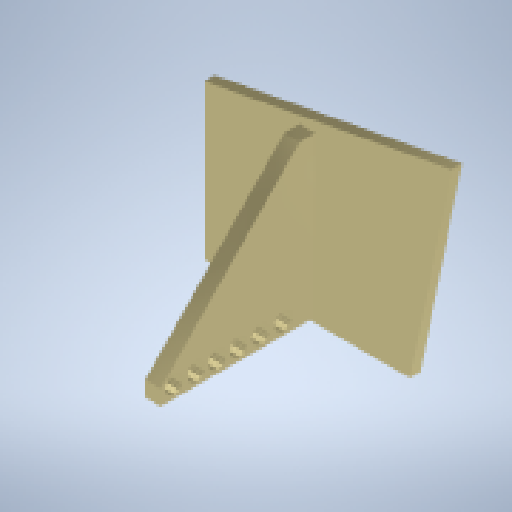
# Autodesk Inventor part: Part5
Saved by Autodesk Inventor 2025.3 (Build 293356000, 356)
## iProperties
Created: 2025-07-14
Part Number: Part5
Material: Generic
Document SubType Name: Modeling
Designer: steve
Density: 1 g/cm^3
Appearance: Default
Author: steve
Autodesk Inventor part; units mm, degrees
ref_plane "YZ Plane" through (0, 0, 0) normal (1, 0, 0) x (0, 1, 0)
ref_plane "XZ Plane" through (0, 0, 0) normal (0, 1, 0) x (-1, 0, 0)
ref_plane "XY Plane" through (0, 0, 0) normal (0, 0, 1) x (1, 0, 0)
sketch "Sketch1" plane through (0, 0, 0) normal (0, 0, 1) x (1, 0, 0)
  line L0 (12.5729, -9.5) -> (10, -7.5)
  line L1 (10, -7.5) -> (-10, -7.5)
  line L2 (-10, -7.5) -> (-10, 7.5)
  line L3 (10, -7.5) -> (14.037, 12.0883)
  line L4 (14.037, 12.0883) -> (-10, 7.5)
  point P0 (0, 0)
  point P1 (-10, 0)
  dimension "d0" = 20
  dimension "d1" = 15
  dimension "d2" = 20
  dimension "d3" = 101.645
  dimension "d18" = 10
  dimension "d19" = 10
  dimension "d20" = 0
  constraints: 10 end point, 1 midpoint, 1 perpendicular
  measures "d0" distance of L0.end L1.end
  measures "d1" distance of L1.end L2.end
  measures "d2" distance of L0.end L3.end
  measures "d3" angle of L3 L1
  measures "d18" distance from line of L2 point (0, 0)
  measures "d19" distance of point (0, 0) point (-10, 0)
  measures "d20" vertical distance of point (0, 0) point (-10, 0)
extrude "Extrusion1" add sketch "Sketch1" along normal blind 1
sketch "Sketch2" plane through (0, 0, 1) normal (0, 0, 1) x (1, 0, 0)
  line L0 (0.75, 5) -> (0.75, -5)
  line L1 (-0.75, -5) -> (-0.75, 5)
  line L2 (-0.75, 5) -> (-0.75, 6.5)
  line L3 (0.75, 6.5) -> (0.75, 5)
  line L4 (-0.75, -5) -> (-0.75, -7)
  line L5 (-0.75, -7) -> (0.75, -7)
  line L6 (0.75, -7) -> (0.75, -5)
  line L7 (-0.75, 6.5) -> (-0.75, 8.5)
  line L8 (-0.75, 8.5) -> (0.75, 8.5)
  line L9 (0.75, 8.5) -> (0.75, 6.5)
  point P0 (0, 0)
  point P1 (0.75, 0)
  dimension "d7" = 10
  dimension "d8" = 1.5
  dimension "d12" = 1.5
  dimension "d21" = 2
  dimension "d22" = 2
  constraints: 20 end point, 4 perpendicular, 3 vertical, 1 midpoint, 1 parallel
  measures "d7" distance of L0.start L0.end
  measures "d8" distance of L1.end L2.end
  measures "d12" distance between parallel lines of L1 L0
  measures "d21" distance of L1.start L4.end
  measures "d22" distance of L2.end L7.end
extrude "Extrusion2" add sketch "Sketch2" along normal blind 15
sketch "Sketch5" plane through (0.75, -7, 1) normal (1, 0, 0) x (0, 0, -1)
  line L0 (0, 15.5) -> (0, 0) projected
  line L1 (0, 15.5) -> (-15, 15.5) projected
  line L2 (-15, 0) -> (-15, 15.5) projected
  line L3 (0, 0) -> (-15, 0) projected
  line L4 (-15, 0) -> (-15, 1.5)
  line L5 (0, 15.5) -> (-1.5, 15.5)
  line L6 (-1.5, 15.5) -> (-15, 1.5)
  line L7 (-15, 1.5) -> (-15, 15.5)
  line L8 (-15, 15.5) -> (-1.5, 15.5)
  point P0 (1, 7)
  dimension "d23" = 1.5
  dimension "d24" = 1.5
  constraints: 10 end point, 2 point on line, 1 collinear, 1 perpendicular
  measures "d23" distance of L2.start L4.end
  measures "d24" distance of L0.start L5.end
extrude "Extrusion4" cut sketch "Sketch5" against normal through all contours L6 L2 L1
sketch "Sketch6" plane through (0.75, -7, 1) normal (1, 0, 0) x (0, 0, -1)
  circle A0 centre (-13.6955, 1.2065) radius 0.86
  circle A1 centre (-11.5498, 1.2065) radius 0.86
  circle A2 centre (-9.5052, 1.2065) radius 0.86
  circle A3 centre (-7.3796, 1.2065) radius 0.86
  circle A4 centre (-5.2541, 1.2065) radius 0.86
  circle A5 centre (-3.0678, 1.2065) radius 0.86
  point P0 (1, 7)
  dimension "d27" = 1.72
  dimension "d28" = 1.72
  dimension "d29" = 1.72
  dimension "d30" = 1.72
  dimension "d31" = 1.72
  dimension "d32" = 1.72
  constraints: 6 centre point
  measures "d27" diameter of A0
  measures "d28" diameter of A1
  measures "d29" diameter of A2
  measures "d30" diameter of A3
  measures "d31" diameter of A4
  measures "d32" diameter of A5
extrude "Extrusion5" cut sketch "Sketch6" against normal through all
body "Solid1"
